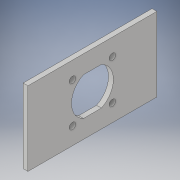
# Autodesk Inventor part: nhk28
Saved by Autodesk Inventor 2019 (Build 230136000, 136)
## iProperties
Created: 2022-02-26
Part Number: nhk28
Material: 一般
Document SubType Name: Sheet Metal
Designer: yuta
Density: 1 g/cm^3
Sheet Metal Rule: Default_mm
Appearance: 既定
Author: yuta
Autodesk Inventor part; units mm, degrees
ref_plane "YZ Plane" through (0, 0, 0) normal (1, 0, 0) x (0, 1, 0)
ref_plane "XZ Plane" through (0, 0, 0) normal (0, 1, 0) x (-1, 0, 0)
ref_plane "XY Plane" through (0, 0, 0) normal (0, 0, 1) x (1, 0, 0)
sketch "スケッチ1" plane through (0, 0, 0) normal (1, 0, 0) x (0, 1, 0)
  line L0 (0, 0) -> (46, 0)
  line L1 (46, 0) -> (46, -80)
  line L2 (46, -80) -> (0, -80)
  line L3 (0, -80) -> (0, 0)
  dimension "d0" = 46
  dimension "d1" = 80
  constraints: 8 end point, 2 parallel, 1 horizontal, 1 perpendicular
  measures "d0" distance of L1.end L2.end
  measures "d1" distance of L0.end L1.end
extrude "押し出し1" add sketch "スケッチ1" along normal blind 3
sketch "スケッチ2" plane through (3, 0, 0) normal (1, 0, 0) x (0, 0, -1)
  circle A0 centre (40, 23) radius 13
  line L0 (34.4379, 34.75) -> (45.5621, 34.75)
  line L1 (34.4379, 11.25) -> (45.5621, 11.25)
  line L2 (80, 46) -> (0, 46) projected
  line L3 (0, 46) -> (0, 0) projected
  dimension "d4" = 26
  dimension "d7" = 23
  dimension "d8" = 40
  dimension "d9" = 23.5
  constraints: 4 end point, 4 point on circle, 1 centre point, 1 horizontal, 1 parallel
  measures "d4" diameter of A0
  measures "d7" distance from line of L2 A0.centre
  measures "d8" distance from line of L3 A0.centre
  measures "d9" distance between parallel lines of L1 L0
extrude "押し出し2" cut sketch "スケッチ2" against normal blind 3 contours A0 L1 L0
sketch "スケッチ3" plane through (3, 0, 0) normal (1, 0, 0) x (0, 0, -1)
  circle A0 centre (40, 23) radius 17.5 construction
  arc A1 (34.4379, 34.75) -> (34.4379, 11.25) centre (40, 23) ccw projected
  arc A2 (45.5621, 11.25) -> (45.5621, 34.75) centre (40, 23) ccw projected
  line L0 (22.5, 23) -> (57.5, 23) construction
  line L1 (40, 5.5) -> (40, 40.5) construction
  line L2 (40, 23) -> (52.3744, 35.3744) construction
  line L3 (40, 23) -> (57.5, 23) construction
  line L4 (52.3744, 35.3744) -> (27.6256, 10.6256) construction
  line L5 (40, 23) -> (52.3744, 10.6256) construction
  line L6 (27.6256, 35.3744) -> (40, 23) construction
  circle A3 centre (52.3744, 35.3744) radius 2.15
  circle A4 centre (52.3744, 10.6256) radius 2.15
  circle A5 centre (27.6256, 10.6256) radius 2.15
  circle A6 centre (27.6256, 35.3744) radius 2.15
  point P0 (0, 0)
  dimension "d12" = 35
  dimension "d13" = 45
  dimension "d14" = 4.3
  dimension "d15" = 4.3
  dimension "d16" = 4.3
  dimension "d17" = 4.3
  constraints: 14 end point, 4 centre point, 4 coincident, 2 horizontal, 2 perpendicular, 2 point on line, 1 collinear, 1 equal length, 12 other
  measures "d13" angle of L3 L2
  measures "d14" diameter of A3
  measures "d15" diameter of A4
  measures "d16" diameter of A5
  measures "d17" diameter of A6
hole "穴1" at (3, 35.3744, -27.6256) at (3, 35.3744, -52.3744) at (3, 10.6256, -52.3744) at (3, 10.6256, -27.6256) direction (-1, 0, 0) diameter 4 depth 3
equation "\"BendRadius\" = Thickness"
equation "\"BendReliefWidth\" = Thickness"
equation "\"BendReliefDepth\" = 0.5 * Thickness"
equation "\"CornerReliefSize\" = 4 * Thickness"
equation "\"MinimumRemnant\" = 2 * Thickness"
equation "\"TransitionRadius\" = BendRadius"
equation "\"JacobiRadiusSize\" = BendRadius"
equation "\"GapSize\" = Thickness"
equation "\"Thickness\" = 0.5"
